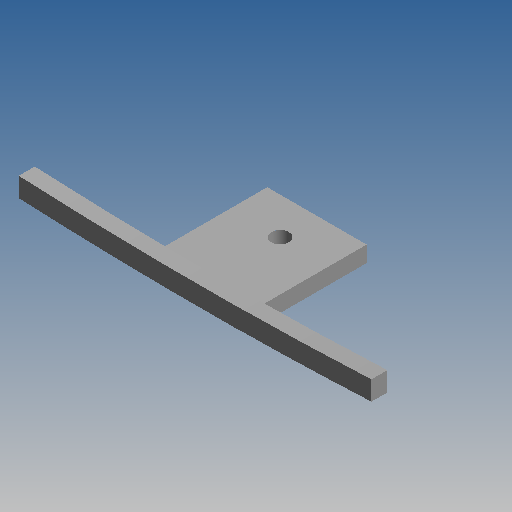
# Autodesk Inventor part: 01-06 Absicherung Box
Saved by Autodesk Inventor 2026.2 (Build 302298000, 298)
## iProperties
Part Number: 01-06 Absicherung Box
Material: Allgemein
Document SubType Name: Modellieren
Designer: Schally
Appearance: Vorgabe
Author: Schally
Autodesk Inventor part; units mm, degrees
ref_plane "YZ-Ebene" through (0, 0, 0) normal (1, 0, 0) x (0, 1, 0)
ref_plane "XZ-Ebene" through (0, 0, 0) normal (0, 1, 0) x (-1, 0, 0)
ref_plane "XY-Ebene" through (0, 0, 0) normal (0, 0, 1) x (1, 0, 0)
sketch "Skizze1" plane through (0, 0, 0) normal (0, 1, 0) x (-1, 0, 0)
  line L0 (-15.5, 11.5) -> (15.5, 11.5)
  line L1 (15.5, 11.5) -> (15.5, -11.5)
  line L2 (15.5, -11.5) -> (-15.5, -11.5)
  line L3 (-15.5, -11.5) -> (-15.5, 11.5)
  line L4 (148.7552, 0) -> (-148.7387, 0) projected
  line L5 (0, -18.1) -> (0, 28.1) projected
  line L6 (0, -11.5) -> (0, 11.5)
  circle A0 centre (0, 0) radius 2.75
  dimension "d0" = 23
  dimension "d1" = 31
  dimension "d3" = 5.5
  constraints: 10 end point, 3 midpoint, 2 parallel, 2 point on line, 1 centre point, 1 horizontal, 1 perpendicular, 2 other
  measures "d0" distance of L0.end L1.end
  measures "d1" distance of L0.start L0.end
  measures "d3" diameter of A0
extrude "Extrusion1" add sketch "Skizze1" along normal blind 5 contours L0 L5 A0 L4 L3 | L0 L1 L4 A0 L5 | L4 A0 L5 L2 L3 | L1 L2 L5 A0 L4
sketch "Skizze2" plane through (-15.5, 0, 11.5) normal (0, 0, 1) x (1, 0, 0)
  line L0 (0, 0) -> (31, 0) projected
  line L1 (31, 0) -> (31, 5) projected
  line L2 (0, 5) -> (31, 5) projected
  line L3 (0, 0) -> (0, 5) projected
  line L4 (0, 0) -> (31, 0) projected
  line L5 (31, 0) -> (31, 5) projected
  line L6 (0, 5) -> (31, 5) projected
  line L7 (0, 0) -> (0, 5) projected
  point P0 (15.5, 0)
extrude "Extrusion2" add sketch "Skizze2" along normal blind 10
sketch "Skizze3" plane through (-15.5, 0, 21.5) normal (0, 0, 1) x (1, 0, 0)
  line L0 (0, 0) -> (31, 0) projected
  arc A0 (-90.0082, 12.8816) -> (120.9918, 12.8816) centre (15.4918, 1123.4066) ccw
  line L1 (8.3371, 5.988) -> (1.4088, 5.988)
  line L2 (1.4088, 5.988) -> (1.4088, -0.012)
  line L3 (8.3371, -0.012) -> (1.4088, -0.012)
  line L4 (8.3371, 5.988) -> (8.3371, -0.012)
  line L5 (29.5747, 5.988) -> (22.6465, 5.988)
  line L6 (22.6465, 5.988) -> (22.6465, -0.012)
  line L7 (29.5747, -0.012) -> (22.6465, -0.012)
  line L8 (29.5747, 5.988) -> (29.5747, -0.012)
  line L9 (70.4918, 10.8726) -> (70.4918, -5.7752)
  line L10 (-39.5082, 12.8816) -> (-39.5082, -5.1111)
  arc A1 (-39.5082, 7.3287) -> (70.4918, 7.3287) centre (15.4918, 1123.4066) ccw
  arc A2 (-90.7561, 5.0098) -> (121.7396, 5.0098) centre (15.4918, 1123.4066) ccw
  line L11 (8.3371, 5.988) -> (1.4088, 5.988)
  line L12 (1.4088, 5.988) -> (1.4088, -0.012)
  line L13 (8.3371, -0.012) -> (1.4088, -0.012)
  line L14 (8.3371, 5.988) -> (8.3371, -0.012)
  point P0 (15.5, 0)
  point P1 (15.4918, 5.988)
  point P2 (-39.5082, 6.6061)
  point P3 (70.4918, 1.3214)
  point P4 (-39.5082, 1.3214)
  point P5 (7.8951, 0)
  point P6 (22.6465, 0)
  point P7 (29.5747, 0.0626)
  dimension "d9" = 6
  dimension "d10" = 110
  constraints: 28 end point, 6 point on circle, 4 point on line, 3 centre point, 2 horizontal alignment, 2 vertical
  measures "d9" radial gap between concentric circles of A1 A2
  measures "d10" distance between parallel lines of L9 L10
extrude "Extrusion3" add sketch "Skizze3" along normal blind 5 contours A2 L2 L1 L4 L0 | A2 L10 A1 L9 L8 L5 L6 L0 L4 L1 L2 | L6 L5 L8 A2 L0 | L0 L8 L7 L6 | A2 L8 L0
